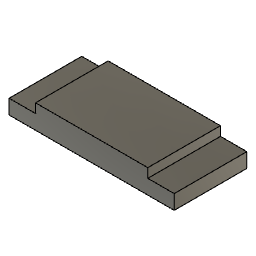
ObudowaWkładka v1 (Autodesk Fusion 360 design; units mm, degrees)
Autodesk Fusion 360 part; units mm, degrees
sketch "Sketch1" plane through (0, 0, 0) normal (0, 0, 1) x (1, 0, 0)
  line L0 (-50, 50) -> (35, 50)
  line L1 (35, 50) -> (35, -5)
  line L2 (35, -5) -> (-50, -5)
  line L3 (-50, -5) -> (-50, 50)
  constraint horizontal L0
  constraint vertical L1
  constraint horizontal L2
  constraint vertical L3
extrude "Extrude1" add sketch "Sketch1" along normal blind 19
extrude "Extrude2" cut 1 faces at (-21.6667, 31.6667, 19) along direction (0, 0, -1) blind 1
sketch "Sketch2" plane through (0, 0, 0) normal (0, 0, 1) x (1, 0, 0)
  line L0 (35, 50) -> (55, 50)
  line L1 (55, 50) -> (55, -5)
  line L2 (55, -5) -> (35, -5)
  line L3 (35, -5) -> (35, 50)
  line L4 (-50, 50) -> (-70, 50)
  line L5 (-70, 50) -> (-70, -5)
  line L6 (-70, -5) -> (-50, -5)
  line L7 (-50, -5) -> (-50, 50)
  constraint horizontal L0
  constraint vertical L1
  constraint horizontal L2
  constraint vertical L3
  constraint horizontal L4
  constraint vertical L5
  constraint horizontal L6
  constraint vertical L7
extrude "Extrude3" add sketch "Sketch2" along normal blind 11
